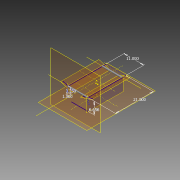
# Autodesk Inventor part: Wheelbase
Saved by Autodesk Inventor 2015 (Build 190159000, 159)
## iProperties
Created: 2016-01-19
Part Number: Wheelbase
Material: Generic
Document SubType Name: Modeling
Designer: sethbattis
Density: 1 g/cm^3
Appearance: Default
Author: sethbattis
Autodesk Inventor part; units mm, degrees
ref_plane "YZ Plane" through (0, 0, 0) normal (1, 0, 0) x (0, 1, 0)
sketch "Dimensions" plane through (0, 0, 0) normal (0, 1, 0) x (-1, 0, 0)
  line L0 (288.9748, 0) -> (-288.9748, 0) construction
  line L1 (0, -373.38) -> (0, 373.38) construction
  line L2 (133.35, 266.7) -> (133.35, -266.7) construction
  line L3 (-133.35, 266.7) -> (-133.35, -266.7) construction
  line L4 (133.35, -266.7) -> (-133.35, -266.7) construction
  line L5 (133.35, 266.7) -> (-133.35, 266.7) construction
  point P0 (0, 0)
  dimension "d61" = 266.7
  dimension "d62" = 533.4
  constraints: 8 coincident, 8 end point, 2 vertical, 1 horizontal, 1 perpendicular, 2 other
  measures "d61" distance of L4.start L4.end
  measures "d62" distance of L3.start L3.end
ref_plane "Kingpin Vertical Plane End C" through (-133.35, 0, 266.7) normal (0, 0, 1) x (1, 0, 0)
sketch "Kingpin Angles" plane through (-133.35, 0, 266.7) normal (0, 0, 1) x (1, 0, 0)
  line L0 (-73.0606, 22.4802) -> (73.0606, -22.4802)
  line L1 (339.7606, 22.4802) -> (193.6394, -22.4802)
  line L2 (38.1, -169.0624) -> (266.7, -169.0624)
  line L3 (0, 0) -> (-25.4, -82.55) construction
  line L4 (-25.4, -82.55) -> (0, -82.55) construction
  line L5 (0, -82.55) -> (0, 0) construction
  line L6 (266.7, 0) -> (292.1, -82.55) construction
  line L7 (292.1, -82.55) -> (266.7, -82.55) construction
  line L8 (266.7, -82.55) -> (266.7, 0) construction
  point P0 (133.35, 0)
  dimension "d67" = 169.0624
  dimension "d70" = 25.4
  dimension "d71" = 82.55
  constraints: 18 end point, 4 perpendicular, 3 equal length, 3 horizontal, 2 midpoint
  measures "d67" distance from line of L2 L6.start
  measures "d70" distance of L3.end L4.end
  measures "d71" distance of L4.end L3.start
ref_plane "Kingpin Tops Side A" through (-206.4106, 22.4802, 266.7) normal (0.2940858, 0.955779, 0) x (0.955779, -0.2940858, 0)
ref_plane "Kingpin Tops Side B" through (60.2894, -22.4802, 266.7) normal (-0.2940858, 0.955779, 0) x (0.955779, 0.2940858, 0)
sketch "Sketch15" plane through (-206.4106, 22.4802, 266.7) normal (0.2940858, 0.955779, 0) x (0.955779, -0.2940858, 0)
  line L0 (76.4409, 0) -> (76.4409, 533.4)
  point P0 (203.894, 266.7)
  constraints: 2 end point, 1 vertical
sketch "Sketch16" plane through (60.2894, -22.4802, 266.7) normal (-0.2940858, 0.955779, 0) x (0.955779, 0.2940858, 0)
  line L0 (76.4409, 0) -> (76.4409, 533.4)
  point P0 (-51.0122, 266.7)
  constraints: 2 end point, 1 vertical
ref_plane "Ground Plane (Dead Ahead)" through (-95.25, -169.0624, 266.7) normal (0, 1, 0) x (1, 0, 0)
sketch "Ground Center" plane through (-95.25, -169.0624, 266.7) normal (0, 1, 0) x (1, 0, 0)
  line L0 (95.25, 640.08) -> (95.25, -106.68) construction
  line L1 (-193.7248, 266.7) -> (384.2248, 266.7) construction
  point P0 (95.25, 266.7)
  point P1 (95.25, 266.7)
  constraints: 1 coincident
ref_plane "Axle Ends" through (133.35, 0, 266.7) normal (-1, 0, 0) x (0, 0, -1)
sketch "Sketch18" plane through (133.35, 0, 266.7) normal (-1, 0, 0) x (0, 0, -1)
  circle A0 centre (0, 0) radius 9.525
  circle A1 centre (484.4419, 0) radius 9.525
  point P0 (266.7, 0)
  dimension "d73" = 19.05
  dimension "d74" = 19.05
  constraints: 2 centre point
  measures "d73" diameter of A0
  measures "d74" diameter of A1
extrude "Axles" add sketch "Sketch18" along normal up to surface (266.7 mm away)
body "Solid6"
